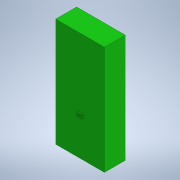
# Autodesk Inventor part: ENGR131 KC Design 2
Saved by Autodesk Inventor 2020 (Build 240168000, 168)
## iProperties
Created: 2019-11-20
Part Number: ENGR131 KC Design 2
Material: Generic
Document SubType Name: Modeling
Designer: camde
Density: 1 g/cm^3
Appearance: Dark Green
Mass: 15619 g
Surface Area: 11687.1 cm^2
Volume: 15619 cm^3
Author: camde
Autodesk Inventor part; units mm, degrees
ref_plane "YZ Plane" through (0, 0, 0) normal (1, 0, 0) x (0, 1, 0)
ref_plane "XZ Plane" through (0, 0, 0) normal (0, 1, 0) x (-1, 0, 0)
ref_plane "XY Plane" through (0, 0, 0) normal (0, 0, 1) x (1, 0, 0)
sketch "Sketch1" plane through (0, 0, 0) normal (0, 0, 1) x (1, 0, 0)
  line L0 (-13.6697, 534.1801) -> (367.3303, 534.1801)
  line L1 (367.3303, 534.1801) -> (367.3303, -10.1056)
  line L2 (367.3303, -10.1056) -> (-13.6697, -10.1056)
  line L3 (-13.6697, -10.1056) -> (-13.6697, 534.1801)
  point P0 (0, 0)
  dimension "d0" = 381
  dimension "d1" = 544.2857
  constraints: 8 end point, 2 parallel, 1 horizontal, 1 perpendicular
  measures "d0" distance of L1.end L2.end
  measures "d1" distance of L2.end L0.start
extrude "Extrusion1" add sketch "Sketch1" along normal blind 163.2857
sketch "Sketch2" plane through (-13.6697, 534.1801, 0) normal (0, 1, 0) x (1, 0, 0)
  line L0 (27.2143, -136.0717) -> (353.786, -136.0717)
  line L1 (353.786, -136.0717) -> (353.786, -27.214)
  line L2 (353.786, -27.214) -> (27.2143, -27.214)
  line L3 (27.2143, -27.214) -> (27.2143, -136.0717)
  line L4 (0, 0) -> (0, -163.2857) projected
  line L5 (381, 0) -> (0, 0) projected
  line L6 (381, 0) -> (381, -163.2857) projected
  line L7 (381, -163.2857) -> (0, -163.2857) projected
  point P0 (13.6697, 0)
  dimension "d4" = 27.2143
  dimension "d5" = 27.214
  dimension "d6" = 27.214
  dimension "d7" = 27.214
  constraints: 8 end point, 2 parallel, 1 horizontal, 1 perpendicular
  measures "d4" distance between parallel lines of L4 L3
  measures "d5" distance between parallel lines of L5 L2
  measures "d6" distance between parallel lines of L6 L1
  measures "d7" distance between parallel lines of L7 L0
extrude "Extrusion2" cut sketch "Sketch2" against normal blind 218.3674 contours L3 L2 L1 L0
sketch "Sketch3" plane through (-13.6697, 315.8127, 0) normal (0, 1, 0) x (1, 0, 0)
  line L0 (353.786, -27.214) -> (353.786, -136.0717) projected
  line L1 (27.2143, -27.214) -> (353.786, -27.214) projected
  line L2 (353.786, -136.0717) -> (209.768, -136.0717)
  line L3 (209.768, -136.0717) -> (209.768, -27.214)
  line L4 (209.768, -27.214) -> (353.786, -27.214)
  line L5 (353.786, -27.214) -> (353.786, -136.0717)
  line L6 (353.786, -136.0717) -> (27.2143, -136.0717) projected
  line L7 (27.2143, -136.0717) -> (171.2323, -136.0717)
  line L8 (171.2323, -136.0717) -> (171.2323, -27.214)
  line L9 (171.2323, -27.214) -> (27.2143, -27.214)
  line L10 (27.2143, -27.214) -> (27.2143, -136.0717)
  point P0 (13.6697, 0)
  point P1 (27.2143, -27.214)
  point P2 (171.2323, -27.214)
  dimension "d10" = 144.018
  dimension "d11" = 144.018
  constraints: 16 end point, 4 parallel, 2 horizontal, 2 perpendicular, 2 point on line
  measures "d10" distance of L3.end L4.end
  measures "d11" distance of L9.end L8.end
extrude "Extrusion3" cut sketch "Sketch3" against normal blind 436.0817 contours L0 L2 L3 L1 | L8 L6 L10 L1
sketch "Sketch4" plane through (-13.6697, 315.8127, 0) normal (0, 1, 0) x (1, 0, 0)
  line L0 (171.2323, -27.214) -> (209.768, -27.214) projected
  line L1 (209.768, -136.0717) -> (209.768, -27.214) projected
  line L2 (171.2323, -27.214) -> (209.768, -27.214)
  line L3 (209.768, -27.214) -> (209.768, -136.0717)
  line L4 (209.768, -136.0717) -> (171.2323, -136.0717)
  line L5 (171.2323, -136.0717) -> (171.2323, -27.214)
  point P0 (13.6697, 0)
  constraints: 8 end point, 2 parallel, 1 horizontal, 1 perpendicular
extrude "Extrusion4" cut sketch "Sketch4" against normal blind 54.4286
sketch "Sketch5" plane through (13.5445, 534.1801, 27.214) normal (0, 0, 1) x (1, 0, 0)
  line L0 (144.018, -272.796) -> (182.5537, -272.796) projected
  line L1 (163.2859, -272.796) -> (163.2859, -37.2995) construction
  circle A0 centre (163.2859, -251.0246) radius 13.6071
  point P0 (-13.5445, -534.1801)
  dimension "d16" = 27.2143
  dimension "d17" = 21.7714
  constraints: 2 end point, 1 centre point, 1 midpoint, 1 point on line, 1 vertical
  measures "d16" diameter of A0
  measures "d17" distance from line of L0 A0.centre
extrude "Extrusion5" cut sketch "Sketch5" along normal mid plane 489.8571
sketch "Sketch6" plane through (-13.6697, 534.1801, 0) normal (0, 1, 0) x (1, 0, 0)
  line L0 (381, -163.2857) -> (0, -163.2857) projected
  line L1 (0, 0) -> (0, -163.2857) projected
  line L2 (27.2143, -163.2857) -> (0, -163.2857)
  line L3 (0, -163.2857) -> (0, 0)
  line L4 (0, 0) -> (26.8469, 0)
  line L5 (27.2143, -27.214) -> (27.2143, -163.2857)
  line L6 (27.2143, -27.214) -> (353.786, -27.214) projected
  line L7 (381, 0) -> (381, -163.2857) projected
  line L8 (27.2143, -27.214) -> (353.786, -27.214)
  line L9 (381, -27.214) -> (381, 0)
  line L10 (381, 0) -> (27.2143, 0)
  line L11 (381, 0) -> (0, 0) projected
  line L12 (381, -163.2857) -> (353.786, -163.2857)
  line L13 (353.786, -163.2857) -> (353.786, -27.214)
  line L14 (353.786, 0) -> (381, 0)
  line L15 (381, 0) -> (381, -163.2857)
  line L16 (27.2143, -27.214) -> (27.2143, -136.0717) projected
  line L17 (27.2143, -163.2857) -> (27.2143, -27.214)
  line L18 (27.2143, -27.214) -> (353.786, -27.214)
  line L19 (353.786, -136.0717) -> (353.786, -27.214) projected
  line L20 (353.786, -27.214) -> (353.786, -163.2857)
  point P0 (13.6697, 0)
  constraints: 28 end point, 5 parallel, 4 perpendicular, 4 point on line, 3 horizontal, 2 collinear
extrude "Extrusion6" add sketch "Sketch6" along normal blind 304.8 contours L0 L13 L6 L5 L1 L4 L11 L10 L7
sketch "Sketch7" plane through (13.5445, -10.1056, 27.214) normal (0, 0, 1) x (1, 0, 0)
  line L0 (-27.2143, 849.0857) -> (0, 849.0857) projected
  line L1 (326.5717, 849.0857) -> (326.5717, 0) projected
  line L2 (0, 849.0857) -> (326.5717, 849.0857)
  line L3 (326.5717, 849.0857) -> (326.5717, 805.1588)
  line L4 (326.5717, 805.1588) -> (0, 805.1588)
  line L5 (0, 805.1588) -> (0, 849.0857)
  point P0 (-13.5445, 10.1056)
  constraints: 8 end point, 2 parallel, 1 horizontal, 1 perpendicular, 1 point on line
extrude "Extrusion7" add sketch "Sketch7" along normal up to surface (136.0717 mm away)
sketch "Sketch8" plane through (13.5445, 534.1801, 163.2857) normal (0, 1, 0) x (1, 0, 0)
  line L0 (0, 27.214) -> (144.018, 27.214) projected
  line L1 (0, 27.214) -> (353.7857, 27.214)
  line L2 (353.7857, 27.214) -> (353.7857, 0)
  line L3 (353.7857, 0) -> (0, 0)
  line L4 (0, 0) -> (0, 27.214)
  point P0 (-13.5445, 163.2857)
  point P1 (144.018, 27.214)
  constraints: 8 end point, 2 parallel, 1 horizontal, 1 perpendicular
extrude "Extrusion8" add sketch "Sketch8" along normal blind 300
sketch "Sketch9" plane through (0, 0, 0) normal (0, 0, -1) x (-1, 0, 0)
  line L0 (-340.3303, 794.9801) -> (-13.3303, 794.9801)
  line L1 (-13.3303, 794.9801) -> (-13.3303, 627.4847)
  line L2 (-340.3303, 794.9801) -> (-340.3303, 627.4847)
  line L3 (-340.3303, 627.4847) -> (-13.3303, 627.4847)
  line L4 (-367.3303, 838.9801) -> (13.6697, 838.9801) projected
  line L5 (13.6697, -10.1056) -> (13.6697, 838.9801) projected
  line L6 (-367.3303, -10.1056) -> (-367.3303, 838.9801) projected
  point P0 (0, 0)
  dimension "d26" = 44
  dimension "d27" = 27
  dimension "d28" = 27
  constraints: 8 end point, 2 perpendicular, 1 horizontal, 1 vertical
  measures "d26" distance between parallel lines of L4 L0
  measures "d27" distance between parallel lines of L5 L1
  measures "d28" distance between parallel lines of L6 L2
extrude "Extrusion9" cut sketch "Sketch9" against normal blind 50
sketch "Sketch10" plane through (0, 0, 0) normal (0, 0, -1) x (-1, 0, 0)
  point P0 (0, 0)
sketch "Sketch11" plane through (340.3303, 627.4847, 0) normal (-1, 0, 0) x (0, 0, 1)
  point P0 (0, -627.4847)
sketch "Sketch12" plane through (0, 0, 163.2857) normal (0, 0, 1) x (1, 0, 0)
  circle A0 centre (176.8304, 283.1555) radius 13.6071 projected
  line L0 (194.8304, 297.5763) -> (176.8304, 297.5763)
  line L1 (194.8304, 297.5763) -> (199.5304, 297.5763)
  line L2 (199.5304, 297.5763) -> (199.5304, 268.7347)
  line L3 (176.8304, 297.5763) -> (152.6961, 297.5763)
  line L4 (152.6961, 297.5763) -> (152.6961, 289.0555)
  line L5 (176.8304, 283.1555) -> (176.8304, 289.0555) construction
  line L6 (176.8304, 289.0555) -> (193.4304, 289.0555)
  line L7 (193.4304, 289.0555) -> (193.4304, 285.8555)
  line L8 (176.8304, 289.0555) -> (152.6961, 289.0555)
  line L9 (176.8304, 283.1555) -> (183.0707, 283.1555) construction
  line L10 (194.8304, 268.7347) -> (176.8304, 268.7347)
  line L11 (176.8304, 268.7347) -> (152.6961, 268.7347)
  line L12 (152.6961, 268.7347) -> (152.6961, 277.2555)
  line L13 (176.8304, 277.2555) -> (193.4304, 277.2555)
  line L14 (176.8304, 277.2555) -> (152.6961, 277.2555)
  line L15 (194.8304, 268.7347) -> (199.5304, 268.7347)
  line L16 (193.4304, 277.2555) -> (193.4304, 285.8555)
  point P0 (0, 0)
  dimension "d35" = 5.9
  constraints: 34 end point, 6 perpendicular, 6 symmetric about line, 3 horizontal, 1 parallel, 1 vertical
  measures "d35" distance of L5.start L5.end
extrude "Extrusion10" add sketch "Sketch12" along normal blind 8.3 contours L6 L8 A0 | A0 L8 L4 L3 L0 L1 L2 L15 L10 L11 L12 L14 L13 L16 L7 L6 | A0 L14 L13
body "Solid1"
